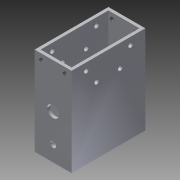
# Autodesk Inventor part: 07
Saved by Autodesk Inventor 2013 (Build 170138000, 138)
## iProperties
Created: 2014-02-11
Material: アルミニウム 6061
Document SubType Name: Modeling
Designer: andou
Density: 2.71 g/cm^3
Mass: 42.5413 g
Surface Area: 167.916 cm^2
Volume: 15.6979 cm^3
Part Number: 07
Author: andou
Title: Long_Serial_Case
Autodesk Inventor part; units mm, degrees
ref_plane "YZ Plane" through (0, 0, 0) normal (1, 0, 0) x (0, 1, 0)
ref_plane "XZ Plane" through (0, 0, 0) normal (0, 1, 0) x (-1, 0, 0)
ref_plane "XY Plane" through (0, 0, 0) normal (0, 0, 1) x (1, 0, 0)
sketch "スケッチ1" plane through (0, 0, 0) normal (0, 0, 1) x (1, 0, 0)
  line L0 (-12.5, 25) -> (12.5, 25)
  line L1 (12.5, 25) -> (12.5, -25)
  line L2 (12.5, -25) -> (-12.5, -25)
  line L3 (-12.5, -25) -> (-12.5, 25)
  line L4 (-10.5, 23) -> (10.5, 23)
  line L5 (10.5, 23) -> (10.5, -23)
  line L6 (10.5, -23) -> (-10.5, -23)
  line L7 (-10.5, -23) -> (-10.5, 23)
  point P0 (0, 0)
  dimension "d0" = 25
  dimension "d1" = 50
  dimension "d2" = 46
  dimension "d3" = 21
  dimension "d4" = 25
  dimension "d5" = 23
  dimension "d6" = 10.5
  dimension "d7" = 12.5
  constraints: 16 end point, 4 parallel, 2 horizontal, 2 perpendicular
  measures "d0" distance of L0.start L0.end
  measures "d1" distance of L2.end L0.start
  measures "d2" distance of L6.end L4.start
  measures "d3" distance of L4.start L4.end
  measures "d4" distance from line of L0 point (0, 0)
  measures "d5" distance from line of point (0, 0) L6
  measures "d6" distance from line of point (0, 0) L7
  measures "d7" distance from line of point (0, 0) L1
extrude "押し出し1" add sketch "スケッチ1" along normal blind 60
sketch "スケッチ2" plane through (-12.5, 25, 0) normal (0, 1, 0) x (1, 0, 0)
  line L0 (0, 0) -> (25, 0) projected
  line L1 (0, 0) -> (0, -60) projected
  arc A0 (6, -33.5) -> (19, -33.5) centre (12.5, -33.5) ccw
  line L2 (6, -33.5) -> (6, 0)
  line L3 (19, -33.5) -> (19, 0)
  point P0 (12.5, 0)
  dimension "d10" = 13
  dimension "d11" = 33.5
  dimension "d12" = 12.5
  constraints: 4 end point, 2 perpendicular, 2 point on circle, 2 point on line, 2 tangent, 1 centre point
  measures "d10" diameter of A0
  measures "d11" distance from line of L0 A0.centre
  measures "d12" distance from line of L1 A0.centre
extrude "押し出し2" cut sketch "スケッチ2" against normal blind 2
sketch "スケッチ3" plane through (-12.5, 25, 60) normal (0, 1, 0) x (1, 0, 0)
  arc A0 (6, 26.5) -> (19, 26.5) centre (12.5, 26.5) ccw projected
  circle A1 centre (4.5, 20) radius 1
  circle A2 centre (4.5, 56) radius 1
  circle A3 centre (20.5, 56) radius 1
  circle A4 centre (20.5, 20) radius 1
  point P0 (12.5, 60)
  dimension "d15" = 6.5
  dimension "d16" = 6.5
  dimension "d17" = 2
  dimension "d18" = 8
  dimension "d19" = 8
  dimension "d20" = 8
  dimension "d21" = 8
  dimension "d22" = 29.5
  dimension "d23" = 29.5
  constraints: 4 centre point, 3 equal radius
  measures "d15" vertical distance of A0.centre A1.centre
  measures "d16" vertical distance of A0.centre A4.centre
  measures "d17" diameter of A1
  measures "d18" horizontal distance of A0.centre A2.centre
  measures "d19" horizontal distance of A0.centre A3.centre
  measures "d20" horizontal distance of A0.centre A4.centre
  measures "d21" horizontal distance of A0.centre A1.centre
  measures "d22" vertical distance of A3.centre A0.centre
  measures "d23" vertical distance of A2.centre A0.centre
hole "穴1" at (-8, 25, 4) at (8, 25, 4) at (8, 25, 40) at (-8, 25, 40) direction (0, -1, 0) diameter 2 depth 2 tip angle 118 counterbore diameter 4 counterbore depth 0.5
sketch "スケッチ4" plane through (-12.5, -25, 0) normal (0, -1, 0) x (1, 0, 0)
  line L0 (25, 0) -> (0, 0) projected
  line L1 (25, 0) -> (25, 60) projected
  circle A0 centre (12.5, 10.5) radius 2
  point P0 (12.5, 0)
  dimension "d31" = 4
  dimension "d32" = 12.5
  dimension "d33" = 10.5
  constraints: 1 centre point
  measures "d31" diameter of A0
  measures "d32" distance from line of A0.centre L1
  measures "d33" distance from line of L0 A0.centre
hole "穴2" at (0, -25, 10.5) direction (0, 1, 0) diameter 4 end through all
sketch "スケッチ5" plane through (-12.5, 25, 60) normal (0, 1, 0) x (1, 0, 0)
  line L0 (0, 0) -> (25, 0) projected
  arc A0 (6, 26.5) -> (19, 26.5) centre (12.5, 26.5) ccw projected
  circle A1 centre (20.5, 4) radius 1.5
  circle A2 centre (4.5, 4) radius 1.5
  point P0 (12.5, 60)
  dimension "d43" = 4
  dimension "d44" = 4
  dimension "d46" = 8
  dimension "d47" = 8
  dimension "d57" = 3
  constraints: 2 centre point, 1 equal radius
  measures "d43" distance from line of A2.centre L0
  measures "d44" distance from line of A1.centre L0
  measures "d46" horizontal distance of A0.centre A2.centre
  measures "d47" horizontal distance of A1.centre A0.centre
  measures "d57" diameter of A2
hole "穴4" at (-8, 25, 56) at (8, 25, 56) direction (0, -1, 0) diameter 3 end through all
thread "ねじ1" size "M3x0.5" class "6H" standard "ANSI Metric M Profile" full length
thread "ねじ2" size "M3x0.5" class "6H" standard "ANSI Metric M Profile" full length
thread "ねじ3" size "M3x0.5" class "6H" standard "ANSI Metric M Profile" full length
thread "ねじ4" size "M3x0.5" class "6H" standard "ANSI Metric M Profile" full length
sketch "スケッチ7" plane through (-12.5, -25, 0) normal (0, -1, 0) x (1, 0, 0)
  line L0 (25, 60) -> (0, 60) projected
  line L1 (25, 0) -> (25, 60) projected
  circle A0 centre (12.5, 30) radius 4
  point P0 (12.5, 0)
  dimension "d78" = 30
  dimension "d79" = 8
  dimension "d80" = 12.5
  constraints: 1 centre point
  measures "d78" distance from line of L0 A0.centre
  measures "d79" diameter of A0
  measures "d80" distance from line of L1 A0.centre
hole "穴5" at (0, -25, 30) direction (0, 1, 0) diameter 8 end through all
sketch "スケッチ8" plane through (12.5, -25, 0) normal (1, 0, 0) x (0, 0, -1)
  line L0 (-60, 50) -> (-60, 0) projected
  line L1 (0, 0) -> (-60, 0) projected
  circle A0 centre (-45, 33) radius 1.5
  circle A1 centre (-45, 17) radius 1.5
  circle A2 centre (-55, 40) radius 1.5
  circle A3 centre (-55, 10) radius 1.5
  line L2 (0, 50) -> (-60, 50) projected
  line L3 (0, 50) -> (0, 0) projected
  point P0 (0, 25)
  dimension "d88" = 16
  dimension "d90" = 3
  dimension "d91" = 15
  dimension "d93" = 17
  dimension "d101" = 30
  dimension "d113" = 10
  dimension "d114" = 15
  dimension "d115" = 5
  dimension "d116" = 5
  dimension "d117" = 60
  constraints: 4 centre point, 3 equal radius
  measures "d88" distance of A0.centre A1.centre
  measures "d90" diameter of A0
  measures "d91" distance from line of A0.centre L0
  measures "d93" distance from line of A1.centre L1
  measures "d101" distance of A2.centre A3.centre
  measures "d113" distance from line of L2 A2.centre
  measures "d114" distance from line of L0 A1.centre
  measures "d115" distance from line of L0 A2.centre
  measures "d116" distance from line of L0 A3.centre
  measures "d117" distance between parallel lines of L3 L0
hole "穴7" at (12.5, 8, 45) at (12.5, -8, 45) at (12.5, -15, 55) at (12.5, 15, 55) direction (-1, 0, 0) diameter 3 end through all
